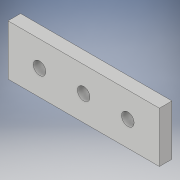
# Autodesk Inventor part: ScissorLiftSliderBracket
Saved by Autodesk Inventor 2018 (Build 220112000, 112)
## iProperties
Created: 2020-01-24
Part Number: ScissorLiftSliderBracket
Material: Generic
Document SubType Name: Modeling
Designer: Cooper
Density: 1 g/cm^3
Appearance: Default
Author: Cooper
Autodesk Inventor part; units mm, degrees
ref_plane "YZ Plane" through (0, 0, 0) normal (1, 0, 0) x (0, 1, 0)
ref_plane "XZ Plane" through (0, 0, 0) normal (0, 1, 0) x (-1, 0, 0)
ref_plane "XY Plane" through (0, 0, 0) normal (0, 0, 1) x (1, 0, 0)
sketch "Sketch1" plane through (0, 0, 0) normal (0, 0, 1) x (1, 0, 0)
  line L0 (0, 0) -> (76.2, 0)
  line L1 (76.2, 0) -> (76.2, 25.4)
  line L2 (76.2, 25.4) -> (0, 25.4)
  line L3 (0, 25.4) -> (0, 0)
  dimension "d0" = 25.4
  dimension "d1" = 76.2
  constraints: 8 end point, 2 parallel, 1 horizontal, 1 perpendicular
  measures "d0" distance of L2.end L0.start
  measures "d1" distance of L1.end L2.end
extrude "Extrusion1" add sketch "Sketch1" along normal blind 6.35
sketch "Sketch2" plane through (0, 0, 6.35) normal (0, 0, 1) x (1, 0, 0)
  line L0 (0, 0) -> (76.2, 0) projected
  line L1 (76.2, 0) -> (76.2, 25.4) projected
  line L2 (76.2, 25.4) -> (0, 25.4) projected
  line L3 (0, 25.4) -> (0, 0) projected
  line L4 (15.875, 12.7) -> (60.325, 12.7) construction
  point P0 (38.1, 12.7)
  point P1 (38.1, 12.7)
  dimension "d4" = 44.45
  dimension "d5" = 12.7
  dimension "d6" = 15.875
  dimension "d14" = 15.875
  constraints: 3 coincident, 2 end point, 1 horizontal, 1 midpoint
  measures "d4" distance of L4.start L4.end
  measures "d5" distance from line of L2 point (15.875, 12.7)
  measures "d6" distance from line of L3 point (15.875, 12.7)
  measures "d14" distance from line of L1 point (60.325, 12.7)
hole "Hole1" at (15.875, 12.7, 6.35) at (38.1, 12.7, 6.35) at (60.325, 12.7, 6.35) direction (0, 0, -1) diameter 6.35 end through all
equation "\"d6\" = d14"
body "Solid1"
